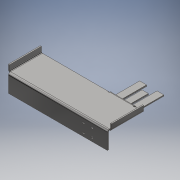
# Autodesk Inventor part: Lamiera supporto pistone taglio
Saved by Autodesk Inventor 2018 (Build 220112000, 112)
## iProperties
Created: 2020-06-15
Part Number: Lamiera supporto pistone taglio
Material: Generico
Document SubType Name: Lamiera
Designer: Francesco
Density: 1 g/cm^3
Sheet Metal Rule: Default_mm
Appearance: Acciaio - Lucido
Author: Francesco
Autodesk Inventor part; units mm, degrees
ref_plane "YZ Plane" through (0, 0, 0) normal (1, 0, 0) x (0, 1, 0)
ref_plane "XZ Plane" through (0, 0, 0) normal (0, 1, 0) x (-1, 0, 0)
ref_plane "XY Plane" through (0, 0, 0) normal (0, 0, 1) x (1, 0, 0)
sketch "Schizzo1" plane through (0, 0, 0) normal (0, 0, 1) x (1, 0, 0)
  line L0 (-225, 72.5) -> (225, 72.5)
  line L1 (225, 72.5) -> (225, -72.5)
  line L2 (225, -72.5) -> (-225, -72.5)
  line L3 (-225, -72.5) -> (-225, 72.5)
  line L4 (-225, 72.5) -> (225, -72.5) construction
  line L5 (225, 72.5) -> (-225, -72.5) construction
  point P0 (0, 0)
  dimension "d0" = 450
  dimension "d1" = 145
  measures "d0" distance of L1.end L2.end
  measures "d1" distance of L0.end L1.end
extrude "Piano1" add sketch "Schizzo1" along normal blind 5
sketch "Schizzo2" plane through (-230, -72.5, 10) normal (-1, 0, 0) x (0, -1, 0)
  line L0 (-145, 0) -> (0, 0)
  line L1 (0, 0) -> (0, 20)
  line L2 (0, 20) -> (-145, 20)
  line L3 (-145, 20) -> (-145, 0)
  constraints: 6 end point, 1 horizontal, 1 perpendicular, 1 vertical
edge flange "Flangia1" height 30 angle 90 thickness 5 bend radius 5 thickness toward (-1, 0, 0) relief straight relief width 5 relief depth 2.5 corner gap 5 corner form 0 edges at (-225, 0, 5) (225, 0, 5) wall of the first edge with corners at (-230, 72.5, 10) (-230, -72.5, 10) (-230, -72.5, 30) (-230, 72.5, 30)
bend "Piega (Bend)1"
corner "Angolo1"
sketch "Schizzo3" plane through (-225, -77.5, -5) normal (0, -1, 0) x (1, 0, 0)
  line L0 (450, 0) -> (0, 0)
  line L1 (0, 0) -> (0, -70)
  line L2 (0, -70) -> (450, -70)
  line L3 (450, -70) -> (450, 0)
  constraints: 6 end point, 1 horizontal, 1 perpendicular, 1 vertical
edge flange "Flangia2" height 80 angle 90 thickness 5 bend radius 5 thickness toward (0, -1, 0) relief straight relief width 5 relief depth 2.5 edges at (0, -72.5, 0) wall of the first edge with corners at (225, -77.5, -5) (-225, -77.5, -5) (-225, -77.5, -75) (225, -77.5, -75)
bend "Piega (Bend)2"
corner "Angolo2"
sketch "Schizzo4" plane through (225, 77.0315, -2.8869) normal (0, 0.9063078, 0.4226183) x (-1, 0, 0)
  line L0 (145, 0) -> (35, 0)
  line L1 (35, 0) -> (35, -17.6293)
  line L2 (35, -17.6293) -> (145, -17.6293)
  line L3 (145, -17.6293) -> (145, 0)
  constraints: 8 end point
edge flange "Flangia3" height 24 angle 65 thickness 5 bend radius 5 thickness toward (0, 0.9063078, 0.4226183) relief straight relief width 5 relief depth 2.5 edges at (0, 72.5, 0) wall of the first edge with corners at (80, 77.0315, -2.8869) (190, 77.0315, -2.8869) (190, 84.482, -18.8645) (80, 84.482, -18.8645)
bend "Piega (Bend)3"
corner "Angolo3"
sketch "Schizzo5" plane through (80, 93.5451, -19.6383) normal (0, 0, -1) x (-1, 0, 0)
  line L0 (-110, 0) -> (0, 0)
  line L1 (0, 0) -> (0, 116.1293)
  line L2 (0, 116.1293) -> (-110, 116.1293)
  line L3 (-110, 116.1293) -> (-110, 0)
  constraints: 6 end point, 1 horizontal, 1 perpendicular, 1 vertical
edge flange "Flangia4" height 122.5 angle 65 thickness 5 bend radius 5 thickness toward (0, 0, -1) relief straight relief width 5 relief depth 2.5 edges at (135, 89.0135, -16.7514) wall of the first edge with corners at (190, 93.5451, -19.6383) (80, 93.5451, -19.6383) (80, 209.6744, -19.6383) (190, 209.6744, -19.6383)
bend "Piega (Bend)4"
corner "Angolo4"
sketch "Schizzo6" plane through (190, 209.6744, -24.6383) normal (0, 0, -1) x (-1, 0, 0)
  line L0 (0, -116.1293) -> (110, -116.1293) projected
  line L1 (110, 0) -> (110, -116.1293) projected
  line L2 (0, -116.1293) -> (0, 0) projected
  line L3 (0, 0) -> (110, 0) projected
  line L4 (77.5, 30) -> (32.5, 30)
  line L5 (32.5, 30) -> (32.5, -30)
  line L6 (32.5, -30) -> (77.5, -30)
  line L7 (77.5, -30) -> (77.5, 30)
  point P0 (190, -209.6744)
  point P1 (55, 0)
  point P2 (55, 30)
  point P3 (77.5, 0)
  dimension "d51" = 45
  dimension "d52" = 60
  constraints: 8 end point, 3 midpoint, 2 parallel, 1 horizontal, 1 horizontal alignment, 1 perpendicular, 1 vertical alignment
  measures "d51" distance of L6.end L5.end
  measures "d52" distance of L5.end L4.end
extrude "Taglia1" cut sketch "Schizzo6" against normal blind 5 contours L5 L4 L7 L3 | L3 L7 L6 L5
sketch "Schizzo7" plane through (-225, -82.5, -75) normal (0, -1, 0) x (1, 0, 0)
  circle A0 centre (379, 16) radius 6.4 projected
  circle A1 centre (341, 16) radius 4.5 projected
  circle A2 centre (379, 54) radius 6.4 projected
  circle A3 centre (341, 54) radius 6.4 projected
  point P0 (225, 75)
  constraints: 4 coincident
hole "Foro1" at (154, -82.5, -59) at (116, -82.5, -59) at (116, -82.5, -21) at (154, -82.5, -21) direction (0, 1, 0) diameter 10 depth 5 tip angle 118
fillet "Arrotondamento angolo1" radius 5 12 edges at (190, 209.6744, -22.1383) (157.5, 209.6744, -22.1383) (157.5, 179.6744, -22.1383) (112.5, 179.6744, -22.1383) (112.5, 209.6744, -22.1383) (80, 209.6744, -22.1383) (232.5, 72.5, 30) (232.5, -72.5, 30) (225, -80, -75) (-232.5, -72.5, 30) (-225, -80, -75) (-232.5, 72.5, 30)
equation "\"d53\" = Spessore"
equation "\"d60\" = Spessore"
equation "\"d2\" = Spessore"
equation "\"d3\" = LarghezzaScaricoPiega"
equation "\"d4\" = ProfonditàScaricoPiega"
equation "\"d5\" = ResiduoMinimo"
equation "\"d6\" = RaggioTransizione"
equation "\"d9\" = RaggioPiega"
equation "\"d10\" = DimensioniScaricoAngolo"
equation "\"d11\" = DimensioneGioco"
equation "\"d12\" = Dimensione_raggio_Jacobi"
equation "\"d13\" = LarghezzaScaricoPiega"
equation "\"d14\" = ProfonditàScaricoPiega"
equation "\"d15\" = ResiduoMinimo"
equation "\"d16\" = RaggioTransizione"
equation "\"d19\" = RaggioPiega"
equation "\"d20\" = DimensioniScaricoAngolo"
equation "\"d21\" = DimensioneGioco"
equation "\"d22\" = Dimensione_raggio_Jacobi"
equation "\"d23\" = LarghezzaScaricoPiega"
equation "\"d24\" = ProfonditàScaricoPiega"
equation "\"d25\" = ResiduoMinimo"
equation "\"d26\" = RaggioTransizione"
equation "\"d29\" = RaggioPiega"
equation "\"d30\" = DimensioniScaricoAngolo"
equation "\"d31\" = DimensioneGioco"
equation "\"d32\" = Dimensione_raggio_Jacobi"
equation "\"d35\" = LarghezzaScaricoPiega"
equation "\"d36\" = ProfonditàScaricoPiega"
equation "\"d37\" = ResiduoMinimo"
equation "\"d38\" = RaggioTransizione"
equation "\"d41\" = RaggioPiega"
equation "\"d42\" = DimensioniScaricoAngolo"
equation "\"d43\" = DimensioneGioco"
equation "\"d44\" = Dimensione_raggio_Jacobi"
equation "\"RaggioPiega\" = Spessore"
equation "\"LarghezzaScaricoPiega\" = Spessore"
equation "\"ProfonditàScaricoPiega\" = 0.5 * Spessore"
equation "\"RaggioTransizione\" = RaggioPiega"
equation "\"Dimensione_raggio_Jacobi\" = RaggioPiega"
equation "\"DimensioneGioco\" = Spessore"
equation "\"Spessore\" = 5"
equation "\"ResiduoMinimo\" = 10"
equation "\"DimensioniScaricoAngolo\" = 20"
